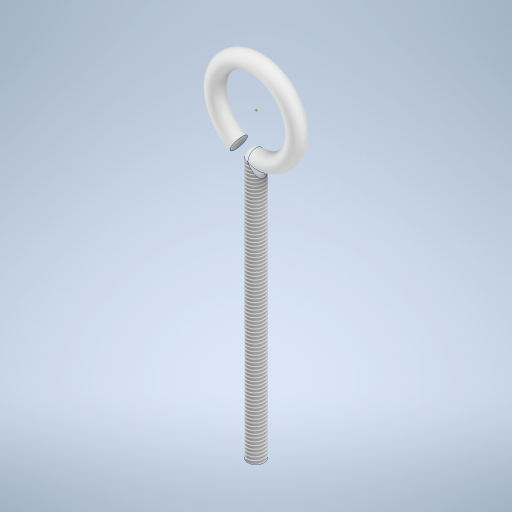
# Autodesk Inventor part: EyeBolt
Saved by Autodesk Inventor 2024 (Build 280153000, 153)
## iProperties
Created: 2023-06-15
Part Number: EyeBolt
Material: Generic
Document SubType Name: Modeling
Designer: 18179
Density: 1 g/cm^3
Appearance: Aluminum - Flat
Author: 18179
Autodesk Inventor part; units mm, degrees
ref_plane "YZ Plane" through (0, 0, 0) normal (1, 0, 0) x (0, 1, 0)
ref_plane "XZ Plane" through (0, 0, 0) normal (0, 1, 0) x (-1, 0, 0)
ref_plane "XY Plane" through (0, 0, 0) normal (0, 0, 1) x (1, 0, 0)
sketch "Sketch1" plane through (0, 0, 0) normal (1, 0, 0) x (0, 1, 0)
  circle A0 centre (0, 0) radius 3.175
  line L0 (3.175, 0) -> (15.875, 0)
  line L1 (15.875, 0) -> (15.875, 11.0604)
  dimension "d0" = 6.35
  dimension "d1" = 12.7
  constraints: 4 end point, 1 coincident, 1 horizontal, 1 horizontal alignment, 1 perpendicular, 2 other
  measures "d1" distance of L0.start L0.end
revolve "Revolution1" add sketch "Sketch1" angle 335 about axis through (0, 15.875, 0) along (0, 0, 1)
sketch "Sketch2" plane through (0, 0, 0) normal (0, 1, 0) x (-1, 0, 0)
  circle A0 centre (0, 0) radius 3.175
  line L0 (15.875, -3.175) -> (-15.875, -3.175) projected
  constraints: 1 centre point, 1 coincident, 1 tangent
extrude "Extrusion1" add sketch "Sketch2" against normal blind 101.6
sketch "Sketch3" plane through (0, 0, 0) normal (0, 1, 0) x (1, 0, 0)
  line L0 (0, 3.175) -> (0, -3.175) projected
  arc A0 (0, 3.175) -> (0, -3.175) centre (0, 0) ccw projected
revolve "Revolution2" add sketch "Sketch3" angle 360 about axis through (0, 0, -3.175) along (0, 0, 1)
fillet "Fillet1" radius 3.175 1 edges at (3.175, -2.9086, 0)
thread "Thread1" size "1/4-20 UNC" class "2A" standard "ANSI Unified Screw Threads" full length
body "Solid1"
